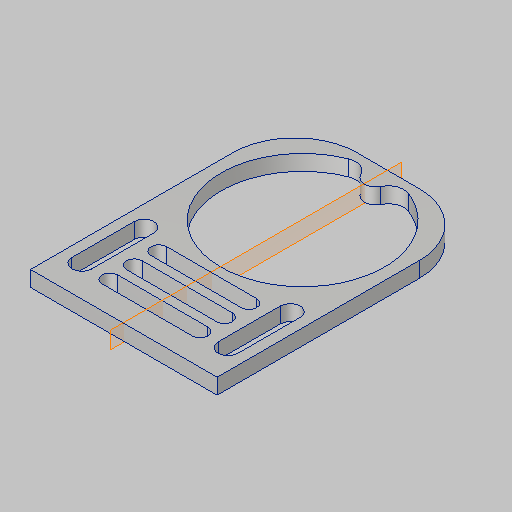
# Autodesk Inventor part: EL2-018
Saved by Autodesk Inventor 2023.5 (Build 275446000, 446)
## iProperties
Created: 2025-01-21
Part Number: EL2-018
Material: Aluminum 6061
Document SubType Name: Modeling
Designer: slick
Density: 2.7 g/cm^3
Appearance: Aluminum - Flat
Author: slick
Autodesk Inventor part; units mm, degrees
ref_plane "XZ Plane" through (0, 0, 0) normal (0, 1, 0) x (-1, 0, 0)
ref_plane "XY Plane" through (0, 0, 0) normal (0, 0, 1) x (1, 0, 0)
sketch "Sketch1" plane through (0, 0, 0) normal (0, 1, 0) x (-1, 0, 0)
  line L0 (-9.2075, -1.5875) -> (9.2075, -1.5875)
  line L1 (9.2075, -1.5875) -> (9.2075, 1.5875)
  line L2 (9.2075, 1.5875) -> (-9.2075, 1.5875)
  line L3 (-9.2075, 1.5875) -> (-9.2075, -1.5875)
  line L4 (-9.2075, -1.5875) -> (9.2075, 1.5875) construction
  line L5 (9.2075, -1.5875) -> (-9.2075, 1.5875) construction
  line L6 (-9.2075, -6.5875) -> (9.2075, -6.5875)
  line L7 (9.2075, -6.5875) -> (9.2075, -3.4125)
  line L8 (9.2075, -3.4125) -> (-9.2075, -3.4125)
  line L9 (-9.2075, -3.4125) -> (-9.2075, -6.5875)
  line L10 (-9.2075, -6.5875) -> (9.2075, -3.4125) construction
  line L11 (9.2075, -6.5875) -> (-9.2075, -3.4125) construction
  line L12 (-9.2075, -11.5875) -> (9.2075, -11.5875)
  line L13 (9.2075, -11.5875) -> (9.2075, -8.4125)
  line L14 (9.2075, -8.4125) -> (-9.2075, -8.4125)
  line L15 (-9.2075, -8.4125) -> (-9.2075, -11.5875)
  line L16 (-9.2075, -11.5875) -> (9.2075, -8.4125) construction
  line L17 (9.2075, -11.5875) -> (-9.2075, -8.4125) construction
  line L18 (19.05, 6.35) -> (-19.05, 6.35)
  line L19 (-19.05, 6.35) -> (-19.05, -47.625)
  line L20 (-19.05, -47.625) -> (19.05, -47.625)
  line L21 (19.05, -47.625) -> (19.05, 6.35)
  circle A0 centre (0, -30.1625) radius 16.6687
  circle A1 centre (9.2075, 0) radius 1.5875
  circle A2 centre (9.2075, -5) radius 1.5875
  circle A3 centre (9.2075, -10) radius 1.5875
  circle A4 centre (-9.2075, -10) radius 1.5875
  circle A5 centre (-9.2075, -5) radius 1.5875
  circle A6 centre (-9.2075, 0) radius 1.5875
  line L22 (14.9225, 0) -> (14.9225, -12.7) construction
  line L23 (12.9032, 0) -> (12.9032, -12.7)
  line L24 (16.9418, -12.7) -> (16.9418, 0)
  arc A7 (16.9418, 0) -> (12.9032, 0) centre (14.9225, 0) ccw
  arc A8 (12.9032, -12.7) -> (16.9418, -12.7) centre (14.9225, -12.7) ccw
  line L25 (-14.9225, 0) -> (-14.9225, -12.7) construction
  line L26 (-16.9418, 0) -> (-16.9418, -12.7)
  line L27 (-12.9032, -12.7) -> (-12.9032, 0)
  arc A9 (-12.9032, 0) -> (-16.9418, 0) centre (-14.9225, 0) ccw
  arc A10 (-16.9418, -12.7) -> (-12.9032, -12.7) centre (-14.9225, -12.7) ccw
  line L28 (10.795, 0) -> (19.05, 0) construction
  line L29 (-10.795, 0) -> (-19.05, 0) construction
  point P0 (0, 0)
  point P1 (0, -5)
  point P2 (0, -10)
  point P3 (0, 6.35)
  point P4 (-9.2075, -11.5875)
  point P5 (9.2075, -8.4125)
  point P6 (-9.2075, -1.5875)
  point P7 (9.2075, 1.5875)
  point P8 (-9.2075, -6.5875)
  point P9 (9.2075, -3.4125)
  point P10 (14.9225, -6.35)
  point P11 (-14.9225, -6.35)
  point P12 (14.9225, 0)
  point P13 (-14.9225, 0)
  dimension "d0" = 18.415
  dimension "d1" = 3.175
  dimension "d6" = 5
  dimension "d7" = 5
  dimension "d8" = 38.1
  dimension "d9" = 53.975
  dimension "d10" = 6.35
  dimension "d11" = 33.3375
  dimension "d20" = 17.4625
  dimension "d21" = 4.0386
  dimension "d22" = 4.0386
  dimension "d23" = 12.7
  dimension "d26" = 12.7
  constraints: 64 end point, 17 midpoint, 12 point on circle, 11 parallel, 8 tangent, 7 centre point, 6 perpendicular, 6 vertical alignment, 5 horizontal alignment, 4 equal length, 4 horizontal, 3 coincident, 2 point on line, 1 vertical, 12 other
  measures "d0" distance of L2.end L1.end
  measures "d1" distance of L1.end L0.end
  measures "d6" distance of point (9.207, -5) point (9.207, 0)
  measures "d7" distance of point (9.207, -10) point (9.207, -5)
  measures "d8" distance between parallel lines of L19 L21
  measures "d9" distance of L20.end L18.start
  measures "d10" distance from line of L18 point (0, 0)
  measures "d11" diameter of A0
  measures "d20" distance from line of L20 A0.centre
  measures "d21" diameter of A8
  measures "d22" diameter of A10
  measures "d23" distance of L25.start L25.end
  measures "d26" distance from line of L18 point (14.922, -6.35)
extrude "Extrusion1" add sketch "Sketch1" along normal blind 3.175
sketch "Sketch2" plane through (0, 3.175, 0) normal (0, 1, 0) x (1, 0, 0)
  circle A0 centre (0, 45.085) radius 2.286
  line L0 (19.05, 47.625) -> (-19.05, 47.625) projected
  point P0 (0, 0)
  point P1 (0, 47.625)
  dimension "d14" = 4.572
  dimension "d15" = 2.54
  constraints: 1 centre point, 1 midpoint
  measures "d14" diameter of A0
  measures "d15" distance of point (0, 47.625) A0.centre
extrude "Extrusion2" add sketch "Sketch2" against normal blind 3.175
fillet "Fillet1" radius 3.175 2 edges at (-1.5575, 1.5875, -46.7583) (1.5575, 1.5875, -46.7583)
fillet "Fillet2" radius 12.7 2 edges at (-19.05, 1.5875, -47.625) (19.05, 1.5875, -47.625)
equation "\"d21\" = d22"
body "Solid1"
